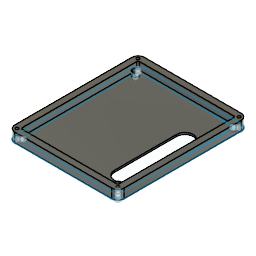
Enclosure_pad (Autodesk Fusion 360 design; units mm, degrees)
part number: 2026-07-29-08-35-26-232
Autodesk Fusion 360 part; units mm, degrees
sketch "Enclosure+pad" plane through (0, 0, 0) normal (0, 0, 1) x (1, 0, 0)
  line L0 (79.9283, 77.1478) -> (79.9283, -54.3522)
  line L1 (-28.5717, 77.1478) -> (78.4283, 77.1478)
  line L2 (-30.0717, -54.3522) -> (-30.0717, 75.6478)
  line L3 (78.4283, -55.8522) -> (-28.5717, -55.8522)
  line L4 (86.9283, -55.8522) -> (86.9283, 77.1478)
  arc A0 (86.9283, 77.1478) -> (79.9283, 84.1478) centre (79.9283, 77.1478) ccw
  arc A1 (79.9283, -62.8522) -> (86.9283, -55.8522) centre (79.9283, -55.8522) ccw
  line L5 (-30.0717, -62.8522) -> (79.9283, -62.8522)
  arc A2 (-30.0717, 84.1478) -> (-37.0717, 77.1478) centre (-30.0717, 77.1478) ccw
  arc A3 (-37.0717, -55.8522) -> (-30.0717, -62.8522) centre (-30.0717, -55.8522) ccw
  line L6 (79.9283, 84.1478) -> (-30.0717, 84.1478)
  line L7 (-37.0717, 77.1478) -> (-37.0717, -55.8522)
  line L8 (79.9283, 75.6478) -> (79.9283, 22.183)
  line L9 (55.1916, 77.1478) -> (79.9283, 77.1478)
  circle A4 centre (-32.3322, 79.3113) radius 1.6
  circle A5 centre (-32.3322, -58.0158) radius 1.6
  circle A6 centre (82.1884, 79.3113) radius 1.6
  circle A7 centre (82.1884, -58.0158) radius 1.6
  circle A8 centre (-26.0717, 70.1478) radius 1.5875
  circle A9 centre (74.9283, -50.8522) radius 1.5875
  arc A10 (-28.5717, 77.1478) -> (-30.0717, 75.6478) centre (-28.5717, 75.6478) ccw
  arc A11 (-30.0717, -54.3522) -> (-28.5717, -55.8522) centre (-28.5717, -54.3522) ccw
  arc A12 (78.4283, -55.8522) -> (79.9283, -54.3522) centre (78.4283, -54.3522) ccw
  arc A13 (79.9283, 75.6478) -> (78.4283, 77.1478) centre (78.4283, 75.6478) ccw
  dimension "d1" = 1.5
  constraint tangent L1 A10
  constraint tangent L2 A10
  constraint tangent L2 A11
  constraint tangent L3 A11
  constraint equal A10 A11
  constraint tangent L0 A12
  constraint tangent L3 A12
  constraint equal A10 A12
  constraint coincident L0.start L1
  constraint coincident L0.start L8
  constraint tangent L1 A13
  constraint tangent L8 A13
  constraint equal A10 A13
  measures "d1" radius of A10
extrude "Extrude6" add sketch "Enclosure+pad" along normal blind 10 contours L0 L9 A13 | L4 A0 A1 L5 A2 A3 L6 L7
extrude "Extrude7" add sketch "Enclosure+pad" along normal blind 2 contours L0 L1 L2 L3 L8 L9 A10 A11 A12 A13 | A8 | A9
sketch "Sketch3" plane through (0, 0, 0) normal (0, 0, -1) x (1, 0, 0)
  circle A0 centre (82.1884, 58.0158) radius 1.6
  circle A1 centre (-32.3322, -79.3113) radius 1.6
  circle A2 centre (82.1884, -79.3113) radius 1.6
  circle A3 centre (-32.3322, 58.0158) radius 1.6
  line L0 (-37.0717, 55.8522) -> (-37.0717, -77.1478)
  arc A4 (-37.0717, -77.1478) -> (-30.0717, -84.1478) centre (-30.0717, -77.1478) ccw
  line L1 (-30.0717, -84.1478) -> (79.9283, -84.1478)
  arc A5 (79.9283, -84.1478) -> (86.9283, -77.1478) centre (79.9283, -77.1478) ccw
  line L2 (86.9283, -77.1478) -> (86.9283, 55.8522)
  arc A6 (86.9283, 55.8522) -> (79.9283, 62.8522) centre (79.9283, 55.8522) ccw
  line L3 (79.9283, 62.8522) -> (-30.0717, 62.8522)
  arc A7 (-30.0717, 62.8522) -> (-37.0717, 55.8522) centre (-30.0717, 55.8522) ccw
  circle A8 centre (82.1884, -79.3113) radius 1.6
  circle A9 centre (82.1884, -79.3113) radius 2.75
  circle A10 centre (82.1884, 58.0158) radius 1.6
  circle A11 centre (82.1884, 58.0158) radius 2.75
  circle A12 centre (-32.3322, 58.0158) radius 1.6
  circle A13 centre (-32.3322, 58.0158) radius 2.75
  circle A14 centre (-32.3322, -79.3113) radius 1.6
  circle A15 centre (-32.3322, -79.3113) radius 2.75
  point P0 (-32.3322, 58.0158)
  dimension "d20" = 5.5
  dimension "d21" = 5.5
  dimension "d22" = 5.5
  dimension "d23" = 5.5
  constraint concentric A8 A9
  constraint concentric A10 A11
  constraint coincident P0 A3.centre
  constraint concentric A14 A15
  measures "d20" diameter of A9
  measures "d21" diameter of A11
  measures "d22" diameter of A13
  measures "d23" diameter of A15
extrude "Extrude8" cut sketch "Sketch3" against normal blind 3 contours A9 | A11 | A13 | A15
extrude "Extrude9" add 1 faces at (-34.7384, 32.3144, 10) along direction (0, 0, 1) blind 0.5
sketch "Sketch4" plane through (0, 0, 2) normal (0, 0, 1) x (-1, 0, 0)
  line L0 (-79.9283, 54.3522) -> (-79.9283, -75.6478)
  arc A0 (-79.9283, -75.6478) -> (-78.4283, -77.1478) centre (-78.4283, -75.6478) ccw
  line L1 (-78.4283, -77.1478) -> (28.5717, -77.1478)
  arc A1 (28.5717, -77.1478) -> (30.0717, -75.6478) centre (28.5717, -75.6478) ccw
  line L2 (30.0717, -75.6478) -> (30.0717, 54.3522)
  arc A2 (30.0717, 54.3522) -> (28.5717, 55.8522) centre (28.5717, 54.3522) ccw
  line L3 (28.5717, 55.8522) -> (-78.4283, 55.8522)
  arc A3 (-78.4283, 55.8522) -> (-79.9283, 54.3522) centre (-78.4283, 54.3522) ccw
  circle A4 centre (26.0717, -70.1478) radius 1.5875
  circle A5 centre (-74.9283, 50.8522) radius 1.5875
  circle A6 centre (26.0717, -70.1478) radius 2.45
  circle A7 centre (26.0717, -70.1478) radius 3.45
  circle A8 centre (-74.9283, 50.8522) radius 2.45
  circle A9 centre (-74.9283, 50.8522) radius 3.45
  point P0 (26.0717, -70.1478)
  dimension "d28" = 4.9
  dimension "d29" = 1
  dimension "d30" = 4.9
  dimension "d31" = 1
  constraint coincident P0 A4.centre
  constraint concentric A5 A8
  measures "d28" diameter of A6
  measures "d30" diameter of A8
extrude "Extrude10" add sketch "Sketch4" along normal blind 4 contours A7 | A9
extrude "Extrude11" add 2 faces at (71.8336, -50.5591, 6) (-23.0553, 69.3967, 6) along direction (0, 0, 1) blind 1
extrude "Extrude12" cut 2 faces at (-23.0553, 69.3967, 7) (71.8336, -50.5591, 7) along direction (0, 0, -1) blind 0.5
sketch "Sketch5" plane through (0, 0, 0) normal (0, 0, 1) x (1, 0, 0)
  line L0 (55.5857, 35) -> (55.5857, -35.6301)
  arc A0 (55.5857, -35.6301) -> (74.4143, -35.6301) centre (65, -35.6301) ccw
  line L1 (74.4143, -35.6301) -> (74.4143, 35)
  arc A1 (74.4143, 35) -> (55.5857, 35) centre (65, 35) ccw
  line L2 (65, 35) -> (65, -35.6301) construction
  constraint tangent L0 A0
  constraint tangent A0 L1
  constraint parallel L0 L1
  constraint tangent L1 A1
  constraint tangent L0 A1
  constraint vertical L2
extrude "Extrude13" cut sketch "Sketch5" along normal blind 70
extrude "Extrude1" [rolled back] along distance 10 taper angle 0
extrude "Extrude2" [rolled back] along distance 2 taper angle 0
sketch "Sketch2" plane through (0, 0, 0) normal (0, 0, 1) x (1, 0, 0)
  circle A0 centre (-32.3322, -58.0158) radius 1.6
  circle A1 centre (-32.3322, 79.3113) radius 1.6
  circle A2 centre (82.1884, 79.3113) radius 1.6
  circle A3 centre (82.1884, -58.0158) radius 1.6
  circle A4 centre (82.1884, 79.3113) radius 2.75
  circle A5 centre (82.1884, -58.0158) radius 2.75
  circle A6 centre (-32.3322, -58.0158) radius 2.75
  circle A7 centre (-32.3322, 79.3113) radius 2.75
  dimension "d8" = 5.5
  dimension "d9" = 5.5
  dimension "d10" = 5.5
  dimension "d11" = 5.5
  constraint concentric A2 A4
  constraint concentric A3 A5
  constraint concentric A0 A6
  constraint concentric A1 A7
  measures "d8" diameter of A4
  measures "d9" diameter of A5
  measures "d10" diameter of A6
  measures "d11" diameter of A7
extrude "Extrude3" [rolled back] along distance 2 taper angle 0
extrude "Extrude4" [rolled back] along distance 3 taper angle 0
extrude "Extrude5" [rolled back] along distance 2 taper angle 0
